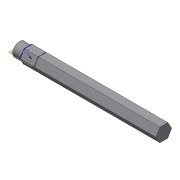
# Autodesk Inventor part: LongShaft
Saved by Autodesk Inventor 2013 SP1 (Build 170176100, 176)
## iProperties
Created: 2013-11-18
Part Number: LongShaft
Material: Generic
Document SubType Name: Modeling
Designer: robotics
Density: 1 g/cm^3
Author: robotics
Autodesk Inventor part; units mm, degrees
ref_plane "YZ Plane" through (0, 0, 0) normal (1, 0, 0) x (0, 1, 0)
ref_plane "XZ Plane" through (0, 0, 0) normal (0, 1, 0) x (-1, 0, 0)
ref_plane "XY Plane" through (0, 0, 0) normal (0, 0, 1) x (1, 0, 0)
sketch "Sketch1" plane through (0, 0, 0) normal (1, 0, 0) x (0, 1, 0)
  line L0 (7.3323, 0) -> (3.6662, -6.35)
  line L1 (3.6662, -6.35) -> (-3.6662, -6.35)
  line L2 (-3.6662, -6.35) -> (-7.3323, 0)
  line L3 (-7.3323, 0) -> (-3.6662, 6.35)
  line L4 (-3.6662, 6.35) -> (3.6662, 6.35)
  line L5 (3.6662, 6.35) -> (7.3323, 0)
  circle A0 centre (0, 0) radius 6.35
  dimension "d0" = 12.7
  constraints: 12 end point, 2 coincident, 1 centre point, 1 horizontal alignment, 1 tangent, 13 other
  measures "d0" diameter of A0
extrude "Extrusion1" add sketch "Sketch1" along normal blind 26.2984
extrude "Extrusion2" add sketch "Sketch1" against normal blind 7.9248 contours A0
ref_plane "Work Plane1" through (0, 7.3323, 0) normal (0, 0, -1) x (1, 0, 0)
sketch "Sketch2" plane through (0, 7.3323, 0) normal (0, 0, -1) x (1, 0, 0)
  line L0 (0, 13.6823) -> (-7.9248, 13.6823) projected
  line L1 (0, 10.9985) -> (0, 14.6647) projected
  line L2 (0, 14.6647) -> (26.2984, 14.6647) projected
  line L3 (12.8618, 14.6647) -> (13.6492, 14.6647)
  line L4 (13.6492, 14.6647) -> (13.6492, 13.6823)
  line L5 (13.6492, 13.6823) -> (12.8618, 13.6823)
  line L6 (12.8618, 13.6823) -> (12.8618, 14.6647)
  line L7 (0, 7.3323) -> (26.2984, 7.3323)
  line L8 (26.2984, 3.6662) -> (26.2984, 10.9985) projected
  line L9 (26.2984, 14.6647) -> (26.2984, 10.9985) projected
  dimension "d7" = 0.7874
  dimension "d9" = 12.6492
  constraints: 10 end point, 2 parallel, 2 perpendicular, 1 collinear, 1 horizontal, 1 midpoint, 1 point on line
  measures "d7" distance between parallel lines of L6 L4
  measures "d9" distance between parallel lines of L9 L4
revolve "Revolution1" cut sketch "Sketch2" angle 360 about axis through (0, 0, 0) along (1, 0, 0)
sketch "Sketch3" plane through (26.2984, 0, 0) normal (1, 0, 0) x (0, 0, -1)
  line L0 (6.35, 3.6662) -> (0, 7.3323) projected
  line L1 (0, 7.3323) -> (-6.35, 3.6662) projected
  line L2 (-6.35, 3.6662) -> (-6.35, -3.6662) projected
  line L3 (-6.35, -3.6662) -> (0, -7.3323) projected
  line L4 (0, -7.3323) -> (6.35, -3.6662) projected
  line L5 (6.35, -3.6662) -> (6.35, 3.6662) projected
  point P0 (0, 0)
extrude "Extrusion3" add sketch "Sketch3" along normal blind 100
body "Solid1"
